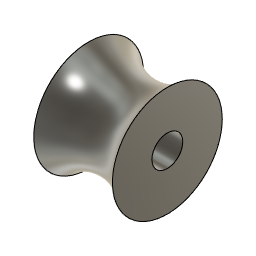
maturita4-kolo v2 (Autodesk Fusion 360 design; units mm, degrees)
Autodesk Fusion 360 part; units mm, degrees
sketch "Sketch1" plane through (0, 0, 0) normal (0, 0, 1) x (1, 0, 0)
  line L0 (0, 0) -> (13, 0)
  line L1 (13, 0) -> (13, 10)
  line L2 (0, 0) -> (0, 10)
  circle A0 centre (6.5, 16) radius 9.5
  line L3 (6.5, 16) -> (6.5, 0)
  dimension "d1" = 13
  dimension "d2" = 10
  dimension "d3" = 10
  dimension "d4" = 19
  dimension "d5" = 16
  constraint coincident L0.start L2.start
  constraint horizontal L0
  constraint perpendicular L0 L1
  constraint perpendicular L0 L2
  constraint coincident A0.centre L3.start
  constraint midpoint L0 L3.end
  measures "d1" distance of L0.start L0.end
  measures "d2" distance of L0.end L1.end
  measures "d3" distance of L0.start L2.end
  measures "d4" diameter of A0
  measures "d5" distance of A0.centre L3.end
revolve "Revolve1" add sketch "Sketch1" angle 360 about axis through (0, 0, 0) along (1, 0, 0) contours L0 L2 A0 L3 | L0 L1 A0 L3
hole "Hole1" at (13, 0, 0) direction (-1, 0, 0) diameter 5.1 depth 13 tip angle 180
